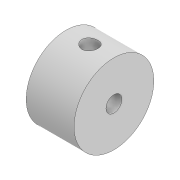
# Autodesk Inventor part: 지름 니플
Saved by Autodesk Inventor 2020 (Build 240168000, 168)
## iProperties
Created: 2020-06-01
Part Number: 지름 니플
Material: 일반
Document SubType Name: Modeling
Designer: Miji
Density: 1 g/cm^3
Appearance: 기본값
Author: Miji
Autodesk Inventor part; units mm, degrees
ref_plane "YZ Plane" through (0, 0, 0) normal (1, 0, 0) x (0, 1, 0)
ref_plane "XZ Plane" through (0, 0, 0) normal (0, 1, 0) x (-1, 0, 0)
ref_plane "XY Plane" through (0, 0, 0) normal (0, 0, 1) x (1, 0, 0)
sketch "스케치1" plane through (0, 0, 0) normal (1, 0, 0) x (0, 1, 0)
  circle A0 centre (0, 0) radius 2.5
  circle A1 centre (0, 0) radius 1
  dimension "d0" = 5
  dimension "d1" = 2
  constraints: 2 centre point, 2 coincident
  measures "d0" diameter of A0
  measures "d1" diameter of A1
extrude "돌출1" add sketch "스케치1" along normal blind 3 contours A0 | A1
sketch "스케치2" plane through (3, 0, 0) normal (1, 0, 0) x (0, 0, -1)
  circle A0 centre (0, 0) radius 0.5
  dimension "d4" = 1
  constraints: 1 centre point, 1 coincident
  measures "d4" diameter of A0
extrude "돌출2" cut sketch "스케치2" against normal blind 11.5
sketch "스케치3" plane through (0, 0, 0) normal (0, 1, 0) x (-1, 0, 0)
  line L0 (-3, 2.5) -> (-3, -2.5) projected
  line L1 (0, 2.5) -> (0, -2.5) projected
  line L2 (0, 0) -> (-3, 0)
  circle A0 centre (-1.5, 0) radius 0.5
  dimension "d7" = 1
  constraints: 2 end point, 2 midpoint, 1 centre point
  measures "d7" diameter of A0
extrude "돌출3" cut sketch "스케치3" along normal mid plane 11.5
